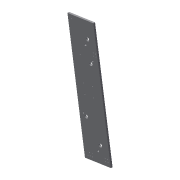
# Autodesk Inventor part: inside wall
Saved by Autodesk Inventor 2020 (Build 240168000, 168)
## iProperties
Created: 2019-10-13
Part Number: inside wall
Material: Generic
Document SubType Name: Modeling
Designer: ball
Density: 1 g/cm^3
Appearance: Default
Author: ball
Autodesk Inventor part; units mm, degrees
ref_plane "YZ Plane" through (0, 0, 0) normal (1, 0, 0) x (0, 1, 0)
ref_plane "XZ Plane" through (0, 0, 0) normal (0, 1, 0) x (-1, 0, 0)
ref_plane "XY Plane" through (0, 0, 0) normal (0, 0, 1) x (1, 0, 0)
ref_plane "Work Plane1" through (-0.0003, 0.0023, 0) normal (0, 0, 1) x (1, 0, 0)
sketch "Sketch1" plane through (-0.0003, 0.0023, 0) normal (0, 0, 1) x (1, 0, 0)
  circle A0 centre (0.0003, -0.0023) radius 6.3373 construction
  circle A1 centre (-49.0975, 326.5271) radius 6.3373 construction
  circle A2 centre (0.0003, -0.0023) radius 6.4135
  circle A3 centre (-49.0975, 326.5271) radius 6.4135
  circle A4 centre (-49.0975, 326.5271) radius 60.325 construction
  circle A5 centre (0.0003, -0.0023) radius 60.325 construction
  circle A6 centre (0.0003, -0.0023) radius 31.75 construction
  circle A7 centre (-49.0975, 326.5271) radius 31.75 construction
  line L0 (-58.7973, -69.8464) -> (40.3672, -54.9357)
  line L1 (-125.8347, 375.9918) -> (-58.0673, 386.1815)
  circle A8 centre (-54.0299, 68.9302) radius 6.3373 construction
  circle A9 centre (-36.6118, 251.3479) radius 6.3373 construction
  circle A10 centre (-54.0299, 68.9302) radius 6.35
  circle A11 centre (-36.6118, 251.3479) radius 6.35
  line L2 (-82.6344, 131.3852) -> (-87.6899, 165.0073) construction
  line L3 (-58.7973, -69.8464) -> (-125.8347, 375.9918)
  arc A12 (-21.1234, 354.0125) -> (-58.0673, 386.1815) centre (-58.7307, 348.1214) ccw
  line L4 (40.3672, -54.9357) -> (-21.1234, 354.0125)
  point P0 (0.0003, -0.0023)
  dimension "d11" = 120.65
  dimension "d0" = 12.827
  dimension "d3" = 12.827
  dimension "d13" = 120.65
  dimension "d14" = 63.5
  dimension "d16" = 63.5
  dimension "d19" = 12.7
  dimension "d20" = 12.7
  constraints: 10 end point, 8 centre point, 8 coincident, 3 tangent, 2 point on circle, 7 other
  measures "d0" diameter of A2
  measures "d3" diameter of A3
  measures "d13" diameter of A5
  measures "d14" diameter of A6
  measures "d16" diameter of A7
  measures "d19" diameter of A10
  measures "d20" diameter of A11
extrude "Extrusion1" add sketch "Sketch1" along normal blind 6.35
sketch "Sketch2" plane through (-0.0003, 0.0023, 6.35) normal (0, 0, 1) x (1, 0, 0)
  circle A0 centre (-59.5704, 139.9475) radius 1.9685 construction
  circle A1 centre (-64.857, 175.1068) radius 1.9685 construction
  circle A2 centre (-25.7636, 145.0307) radius 1.9685 construction
  circle A3 centre (-31.0502, 180.1901) radius 1.9685 construction
  circle A4 centre (-59.5704, 139.9475) radius 1.778
  circle A5 centre (-64.857, 175.1068) radius 1.778
  circle A6 centre (-25.7636, 145.0307) radius 1.778
  circle A7 centre (-31.0502, 180.1901) radius 1.778
  circle A8 centre (-48.1268, -55.3992) radius 1.778
  line L0 (-58.7973, -69.8464) -> (40.3672, -54.9357) projected
  line L1 (-125.8347, 375.9918) -> (-58.7973, -69.8464) projected
  circle A9 centre (-111.3879, 365.3242) radius 1.778
  line L2 (-58.0673, 386.1815) -> (-125.8347, 375.9918) projected
  circle A10 centre (-77.9428, 262.471) radius 1.778
  point P0 (0.0003, -0.0023)
  point P1 (-26.6702, 390.9025)
  dimension "d24" = 3.556
  dimension "d25" = 3.556
  dimension "d26" = 3.556
  dimension "d27" = 3.556
  dimension "d28" = 3.556
  dimension "d29" = 12.7
  dimension "d30" = 12.7
  dimension "d31" = 3.556
  dimension "d32" = 12.6972
  dimension "d33" = 12.7
  dimension "d34" = 3.556
  dimension "d35" = 30.48
  dimension "d36" = 119.38
  constraints: 7 centre point, 4 coincident
  measures "d24" diameter of A4
  measures "d25" diameter of A5
  measures "d26" diameter of A6
  measures "d27" diameter of A7
  measures "d28" diameter of A8
  measures "d29" distance from line of L0 A8.centre
  measures "d30" distance from line of L1 A8.centre
  measures "d31" diameter of A9
  measures "d32" distance from line of L2 A9.centre
  measures "d33" distance from line of L1 A9.centre
  measures "d34" diameter of A10
  measures "d35" distance from line of L1 A10.centre
  measures "d36" distance from line of L2 A10.centre
extrude "Extrusion2" cut sketch "Sketch2" against normal up to surface (6.35 mm away)
sketch "Sketch3" plane through (-0.0003, 0.0023, 6.35) normal (0, 0, 1) x (1, 0, 0)
  circle A0 centre (-32.2734, 257.2219) radius 3.048 construction
  circle A1 centre (-57.7822, 304.4219) radius 4.25 construction
  circle A2 centre (-59.904, 73.2686) radius 3.048 construction
  circle A3 centre (-8.6844, -22.1075) radius 4.25 construction
  circle A4 centre (-57.7822, 304.4219) radius 4.25
  circle A5 centre (-30.2618, 263.525) radius 3.175
  circle A6 centre (-65.0875, 76.3166) radius 3.048
  circle A7 centre (-8.6844, -22.1075) radius 4.25
  line L0 (40.3672, -54.9357) -> (-21.1234, 354.0125) projected
  line L1 (-58.0673, 386.1815) -> (-125.8347, 375.9918) projected
  arc A8 (-34.3449, 253.3797) -> (-33.8476, 250.0726) centre (-36.6118, 251.3479) ccw projected
  arc A9 (-56.2968, 66.8984) -> (-56.7941, 70.2055) centre (-54.0299, 68.9302) ccw projected
  point P0 (0.0003, -0.0023)
  point P1 (-26.6702, 390.9025)
  dimension "d41" = 12.1771
  dimension "d42" = 6.35
  dimension "d43" = 7.3865
  dimension "d44" = 11.0576
  constraints: 4 centre point, 2 coincident, 2 concentric
  measures "d41" vertical distance of A8.centre A5.centre
  measures "d42" horizontal distance of A8.centre A5.centre
  measures "d43" vertical distance of A6.centre A9.centre
  measures "d44" horizontal distance of A6.centre A9.centre
extrude "Extrusion3" cut sketch "Sketch3" against normal through all
sketch "Sketch4" plane through (-0.0003, 0.0023, 6.35) normal (0, 0, 1) x (1, 0, 0)
  arc A0 (-29.6539, 293.2296) -> (-29.0598, 294.034) centre (-28.4354, 292.9511) ccw construction
  arc A1 (-27.2269, 281.8437) -> (-28.0313, 282.4378) centre (-26.9484, 283.0623) ccw construction
  arc A2 (-15.841, 284.2708) -> (-16.4351, 283.4664) centre (-17.0596, 284.5492) ccw construction
  arc A3 (-18.2681, 295.6566) -> (-17.4637, 295.0625) centre (-18.5465, 294.4381) ccw construction
  circle A4 centre (-26.9484, 283.0623) radius 1.7
  circle A5 centre (-28.4354, 292.9511) radius 1.7
  circle A6 centre (-17.0596, 284.5492) radius 1.7
  circle A7 centre (-18.5465, 294.4381) radius 1.7
  circle A8 centre (-26.9484, 283.0623) radius 1.7
  circle A9 centre (-28.4354, 292.9511) radius 1.7
  circle A10 centre (-17.0596, 284.5492) radius 1.7
  circle A11 centre (-18.5465, 294.4381) radius 1.7
  circle A12 centre (-40.0242, -53.8744) radius 1.7
  circle A13 centre (-41.5111, -43.9856) radius 1.7
  circle A14 centre (-30.1354, -52.3875) radius 1.7
  circle A15 centre (-31.6223, -42.4987) radius 1.7
  circle A16 centre (18.6862, -43.9856) radius 1.7
  circle A17 centre (17.1993, -34.0967) radius 1.7
  circle A18 centre (28.575, -42.4987) radius 1.7
  circle A19 centre (27.0881, -32.6098) radius 1.7
  point P0 (0.0003, -0.0023)
  dimension "d47" = 3.4
  dimension "d48" = 3.4
  dimension "d49" = 3.4
  dimension "d50" = 3.4
  dimension "d51" = 3.4
  dimension "d52" = 3.4
  dimension "d53" = 3.4
  dimension "d54" = 3.4
  dimension "d55" = 3.4
  dimension "d56" = 3.4
  dimension "d57" = 3.4
  dimension "d58" = 3.4
  dimension "d59" = 3.4
  dimension "d60" = 3.4
  dimension "d61" = 3.4
  dimension "d62" = 3.4
  constraints: 16 centre point, 4 coincident
  measures "d47" diameter of A4
  measures "d48" diameter of A5
  measures "d49" diameter of A6
  measures "d50" diameter of A7
  measures "d51" diameter of A8
  measures "d52" diameter of A9
  measures "d53" diameter of A10
  measures "d54" diameter of A11
  measures "d55" diameter of A12
  measures "d56" diameter of A13
  measures "d57" diameter of A14
  measures "d58" diameter of A15
  measures "d59" diameter of A16
  measures "d60" diameter of A17
  measures "d61" diameter of A18
  measures "d62" diameter of A19
extrude "Extrusion4" cut sketch "Sketch4" against normal through all
body "Solid1"
